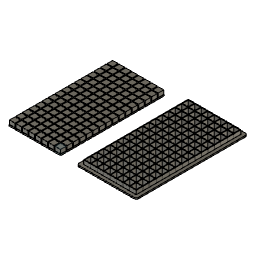
Matriz Altavoz (Autodesk Fusion 360 design; units mm, degrees)
Autodesk Fusion 360 part; units mm, degrees
(part 1 of 2)
sketch "Boceto1" plane through (0, 0, 0) normal (0, 0, 1) x (1, 0, 0)
  line L0 (0, 0) -> (161, 0)
  line L1 (161, 0) -> (161, 81)
  line L2 (161, 81) -> (0, 81)
  line L3 (0, 81) -> (0, 0)
  line L4 (0, 0) -> (0, 1)
  line L5 (0, 1) -> (1, 1)
  line L6 (1, 1) -> (10, 1)
  line L7 (10, 1) -> (10, 10)
  line L8 (10, 10) -> (1, 10)
  line L9 (1, 10) -> (1, 1)
  line L10 (20, 1) -> (20, 10)
  line L11 (20, 10) -> (11, 10)
  line L12 (11, 10) -> (11, 1)
  line L13 (11, 1) -> (20, 1)
  line L14 (30, 1) -> (30, 10)
  line L15 (30, 10) -> (21, 10)
  line L16 (21, 10) -> (21, 1)
  line L17 (21, 1) -> (30, 1)
  line L18 (40, 1) -> (40, 10)
  line L19 (40, 10) -> (31, 10)
  line L20 (31, 10) -> (31, 1)
  line L21 (31, 1) -> (40, 1)
  line L22 (50, 1) -> (50, 10)
  line L23 (50, 10) -> (41, 10)
  line L24 (41, 10) -> (41, 1)
  line L25 (41, 1) -> (50, 1)
  line L26 (60, 1) -> (60, 10)
  line L27 (60, 10) -> (51, 10)
  line L28 (51, 10) -> (51, 1)
  line L29 (51, 1) -> (60, 1)
  line L30 (70, 1) -> (70, 10)
  line L31 (70, 10) -> (61, 10)
  line L32 (61, 10) -> (61, 1)
  line L33 (61, 1) -> (70, 1)
  line L34 (80, 1) -> (80, 10)
  line L35 (80, 10) -> (71, 10)
  line L36 (71, 10) -> (71, 1)
  line L37 (71, 1) -> (80, 1)
  line L38 (90, 1) -> (90, 10)
  line L39 (90, 10) -> (81, 10)
  line L40 (81, 10) -> (81, 1)
  line L41 (81, 1) -> (90, 1)
  line L42 (100, 1) -> (100, 10)
  line L43 (100, 10) -> (91, 10)
  line L44 (91, 10) -> (91, 1)
  line L45 (91, 1) -> (100, 1)
  line L46 (110, 1) -> (110, 10)
  line L47 (110, 10) -> (101, 10)
  line L48 (101, 10) -> (101, 1)
  line L49 (101, 1) -> (110, 1)
  line L50 (120, 1) -> (120, 10)
  line L51 (120, 10) -> (111, 10)
  line L52 (111, 10) -> (111, 1)
  line L53 (111, 1) -> (120, 1)
  line L54 (130, 1) -> (130, 10)
  line L55 (130, 10) -> (121, 10)
  line L56 (121, 10) -> (121, 1)
  line L57 (121, 1) -> (130, 1)
  line L58 (140, 1) -> (140, 10)
  line L59 (140, 10) -> (131, 10)
  line L60 (131, 10) -> (131, 1)
  line L61 (131, 1) -> (140, 1)
  line L62 (150, 1) -> (150, 10)
  line L63 (150, 10) -> (141, 10)
  line L64 (141, 10) -> (141, 1)
  line L65 (141, 1) -> (150, 1)
  line L66 (160, 1) -> (160, 10)
  line L67 (160, 10) -> (151, 10)
  line L68 (151, 10) -> (151, 1)
  line L69 (151, 1) -> (160, 1)
  line L70 (10, 11) -> (10, 20)
  line L71 (10, 20) -> (1, 20)
  line L72 (1, 20) -> (1, 11)
  line L73 (1, 11) -> (10, 11)
  line L74 (20, 11) -> (20, 20)
  line L75 (20, 20) -> (11, 20)
  line L76 (11, 20) -> (11, 11)
  line L77 (11, 11) -> (20, 11)
  line L78 (30, 11) -> (30, 20)
  line L79 (30, 20) -> (21, 20)
  line L80 (21, 20) -> (21, 11)
  line L81 (21, 11) -> (30, 11)
  line L82 (40, 11) -> (40, 20)
  line L83 (40, 20) -> (31, 20)
  line L84 (31, 20) -> (31, 11)
  line L85 (31, 11) -> (40, 11)
  line L86 (50, 11) -> (50, 20)
  line L87 (50, 20) -> (41, 20)
  line L88 (41, 20) -> (41, 11)
  line L89 (41, 11) -> (50, 11)
  line L90 (60, 11) -> (60, 20)
  line L91 (60, 20) -> (51, 20)
  line L92 (51, 20) -> (51, 11)
  line L93 (51, 11) -> (60, 11)
  line L94 (70, 11) -> (70, 20)
  line L95 (70, 20) -> (61, 20)
  line L96 (61, 20) -> (61, 11)
  line L97 (61, 11) -> (70, 11)
  line L98 (80, 11) -> (80, 20)
  line L99 (80, 20) -> (71, 20)
  line L100 (71, 20) -> (71, 11)
  line L101 (71, 11) -> (80, 11)
  line L102 (90, 11) -> (90, 20)
  line L103 (90, 20) -> (81, 20)
  line L104 (81, 20) -> (81, 11)
  line L105 (81, 11) -> (90, 11)
  line L106 (100, 11) -> (100, 20)
  line L107 (100, 20) -> (91, 20)
  line L108 (91, 20) -> (91, 11)
  line L109 (91, 11) -> (100, 11)
  line L110 (110, 11) -> (110, 20)
  line L111 (110, 20) -> (101, 20)
  line L112 (101, 20) -> (101, 11)
  line L113 (101, 11) -> (110, 11)
  line L114 (120, 11) -> (120, 20)
  line L115 (120, 20) -> (111, 20)
  line L116 (111, 20) -> (111, 11)
  line L117 (111, 11) -> (120, 11)
  line L118 (130, 11) -> (130, 20)
  line L119 (130, 20) -> (121, 20)
  line L120 (121, 20) -> (121, 11)
  line L121 (121, 11) -> (130, 11)
  line L122 (140, 11) -> (140, 20)
  line L123 (140, 20) -> (131, 20)
  line L124 (131, 20) -> (131, 11)
  line L125 (131, 11) -> (140, 11)
  line L126 (150, 11) -> (150, 20)
  line L127 (150, 20) -> (141, 20)
  line L128 (141, 20) -> (141, 11)
  line L129 (141, 11) -> (150, 11)
  line L130 (160, 11) -> (160, 20)
  line L131 (160, 20) -> (151, 20)
  line L132 (151, 20) -> (151, 11)
  line L133 (151, 11) -> (160, 11)
  line L134 (10, 21) -> (10, 30)
  line L135 (10, 30) -> (1, 30)
  line L136 (1, 30) -> (1, 21)
  line L137 (1, 21) -> (10, 21)
  line L138 (20, 21) -> (20, 30)
  line L139 (20, 30) -> (11, 30)
  line L140 (11, 30) -> (11, 21)
  line L141 (11, 21) -> (20, 21)
  line L142 (30, 21) -> (30, 30)
  line L143 (30, 30) -> (21, 30)
  line L144 (21, 30) -> (21, 21)
  line L145 (21, 21) -> (30, 21)
  line L146 (40, 21) -> (40, 30)
  line L147 (40, 30) -> (31, 30)
  line L148 (31, 30) -> (31, 21)
  line L149 (31, 21) -> (40, 21)
  line L150 (50, 21) -> (50, 30)
  line L151 (50, 30) -> (41, 30)
  line L152 (41, 30) -> (41, 21)
  line L153 (41, 21) -> (50, 21)
  line L154 (60, 21) -> (60, 30)
  line L155 (60, 30) -> (51, 30)
  line L156 (51, 30) -> (51, 21)
  line L157 (51, 21) -> (60, 21)
  line L158 (70, 21) -> (70, 30)
  line L159 (70, 30) -> (61, 30)
  line L160 (61, 30) -> (61, 21)
  line L161 (61, 21) -> (70, 21)
  line L162 (80, 21) -> (80, 30)
  line L163 (80, 30) -> (71, 30)
  line L164 (71, 30) -> (71, 21)
  line L165 (71, 21) -> (80, 21)
  line L166 (90, 21) -> (90, 30)
  line L167 (90, 30) -> (81, 30)
  line L168 (81, 30) -> (81, 21)
  line L169 (81, 21) -> (90, 21)
  line L170 (100, 21) -> (100, 30)
  line L171 (100, 30) -> (91, 30)
  line L172 (91, 30) -> (91, 21)
  line L173 (91, 21) -> (100, 21)
  line L174 (110, 21) -> (110, 30)
  line L175 (110, 30) -> (101, 30)
  line L176 (101, 30) -> (101, 21)
  line L177 (101, 21) -> (110, 21)
  line L178 (120, 21) -> (120, 30)
  line L179 (120, 30) -> (111, 30)
  line L180 (111, 30) -> (111, 21)
  line L181 (111, 21) -> (120, 21)
  line L182 (130, 21) -> (130, 30)
  line L183 (130, 30) -> (121, 30)
  line L184 (121, 30) -> (121, 21)
  line L185 (121, 21) -> (130, 21)
  line L186 (140, 21) -> (140, 30)
  line L187 (140, 30) -> (131, 30)
  line L188 (131, 30) -> (131, 21)
  line L189 (131, 21) -> (140, 21)
  line L190 (150, 21) -> (150, 30)
  line L191 (150, 30) -> (141, 30)
  line L192 (141, 30) -> (141, 21)
  line L193 (141, 21) -> (150, 21)
  line L194 (160, 21) -> (160, 30)
  line L195 (160, 30) -> (151, 30)
  line L196 (151, 30) -> (151, 21)
  line L197 (151, 21) -> (160, 21)
  line L198 (10, 31) -> (10, 40)
  line L199 (10, 40) -> (1, 40)
  line L200 (1, 40) -> (1, 31)
  line L201 (1, 31) -> (10, 31)
  line L202 (20, 31) -> (20, 40)
  line L203 (20, 40) -> (11, 40)
  line L204 (11, 40) -> (11, 31)
  line L205 (11, 31) -> (20, 31)
  line L206 (30, 31) -> (30, 40)
  line L207 (30, 40) -> (21, 40)
  line L208 (21, 40) -> (21, 31)
  line L209 (21, 31) -> (30, 31)
  line L210 (40, 31) -> (40, 40)
  line L211 (40, 40) -> (31, 40)
  line L212 (31, 40) -> (31, 31)
  line L213 (31, 31) -> (40, 31)
  line L214 (50, 31) -> (50, 40)
  line L215 (50, 40) -> (41, 40)
  line L216 (41, 40) -> (41, 31)
  line L217 (41, 31) -> (50, 31)
  line L218 (60, 31) -> (60, 40)
  line L219 (60, 40) -> (51, 40)
  line L220 (51, 40) -> (51, 31)
  line L221 (51, 31) -> (60, 31)
  line L222 (70, 31) -> (70, 40)
  line L223 (70, 40) -> (61, 40)
  line L224 (61, 40) -> (61, 31)
  line L225 (61, 31) -> (70, 31)
  line L226 (80, 31) -> (80, 40)
  line L227 (80, 40) -> (71, 40)
  line L228 (71, 40) -> (71, 31)
  line L229 (71, 31) -> (80, 31)
  line L230 (90, 31) -> (90, 40)
  line L231 (90, 40) -> (81, 40)
  line L232 (81, 40) -> (81, 31)
  line L233 (81, 31) -> (90, 31)
  line L234 (100, 31) -> (100, 40)
  line L235 (100, 40) -> (91, 40)
  line L236 (91, 40) -> (91, 31)
  line L237 (91, 31) -> (100, 31)
  line L238 (110, 31) -> (110, 40)
  line L239 (110, 40) -> (101, 40)
  line L240 (101, 40) -> (101, 31)
  line L241 (101, 31) -> (110, 31)
  line L242 (120, 31) -> (120, 40)
  line L243 (120, 40) -> (111, 40)
  line L244 (111, 40) -> (111, 31)
  line L245 (111, 31) -> (120, 31)
  line L246 (130, 31) -> (130, 40)
  line L247 (130, 40) -> (121, 40)
  line L248 (121, 40) -> (121, 31)
  line L249 (121, 31) -> (130, 31)
  line L250 (140, 31) -> (140, 40)
  line L251 (140, 40) -> (131, 40)
  line L252 (131, 40) -> (131, 31)
  line L253 (131, 31) -> (140, 31)
  line L254 (150, 31) -> (150, 40)
  line L255 (150, 40) -> (141, 40)
  line L256 (141, 40) -> (141, 31)
  line L257 (141, 31) -> (150, 31)
  line L258 (160, 31) -> (160, 40)
  line L259 (160, 40) -> (151, 40)
  line L260 (151, 40) -> (151, 31)
  line L261 (151, 31) -> (160, 31)
  line L262 (10, 41) -> (10, 50)
  line L263 (10, 50) -> (1, 50)
  line L264 (1, 50) -> (1, 41)
  line L265 (1, 41) -> (10, 41)
  line L266 (20, 41) -> (20, 50)
  line L267 (20, 50) -> (11, 50)
  line L268 (11, 50) -> (11, 41)
  line L269 (11, 41) -> (20, 41)
  line L270 (30, 41) -> (30, 50)
  line L271 (30, 50) -> (21, 50)
  line L272 (21, 50) -> (21, 41)
  line L273 (21, 41) -> (30, 41)
  line L274 (40, 41) -> (40, 50)
  line L275 (40, 50) -> (31, 50)
  line L276 (31, 50) -> (31, 41)
  line L277 (31, 41) -> (40, 41)
  line L278 (50, 41) -> (50, 50)
  line L279 (50, 50) -> (41, 50)
  line L280 (41, 50) -> (41, 41)
  line L281 (41, 41) -> (50, 41)
  line L282 (60, 41) -> (60, 50)
  line L283 (60, 50) -> (51, 50)
  line L284 (51, 50) -> (51, 41)
  line L285 (51, 41) -> (60, 41)
  line L286 (70, 41) -> (70, 50)
  line L287 (70, 50) -> (61, 50)
  line L288 (61, 50) -> (61, 41)
  line L289 (61, 41) -> (70, 41)
  line L290 (80, 41) -> (80, 50)
  line L291 (80, 50) -> (71, 50)
  line L292 (71, 50) -> (71, 41)
  line L293 (71, 41) -> (80, 41)
  line L294 (90, 41) -> (90, 50)
  line L295 (90, 50) -> (81, 50)
  line L296 (81, 50) -> (81, 41)
  line L297 (81, 41) -> (90, 41)
  line L298 (100, 41) -> (100, 50)
  line L299 (100, 50) -> (91, 50)
  line L300 (91, 50) -> (91, 41)
  line L301 (91, 41) -> (100, 41)
  line L302 (110, 41) -> (110, 50)
  line L303 (110, 50) -> (101, 50)
  line L304 (101, 50) -> (101, 41)
  line L305 (101, 41) -> (110, 41)
  line L306 (120, 41) -> (120, 50)
  line L307 (120, 50) -> (111, 50)
  line L308 (111, 50) -> (111, 41)
  line L309 (111, 41) -> (120, 41)
  line L310 (130, 41) -> (130, 50)
  line L311 (130, 50) -> (121, 50)
  line L312 (121, 50) -> (121, 41)
  line L313 (121, 41) -> (130, 41)
  line L314 (140, 41) -> (140, 50)
  line L315 (140, 50) -> (131, 50)
  line L316 (131, 50) -> (131, 41)
  line L317 (131, 41) -> (140, 41)
  line L318 (150, 41) -> (150, 50)
  line L319 (150, 50) -> (141, 50)
  line L320 (141, 50) -> (141, 41)
  line L321 (141, 41) -> (150, 41)
  line L322 (160, 41) -> (160, 50)
  line L323 (160, 50) -> (151, 50)
  line L324 (151, 50) -> (151, 41)
  line L325 (151, 41) -> (160, 41)
  line L326 (10, 51) -> (10, 60)
  line L327 (10, 60) -> (1, 60)
  line L328 (1, 60) -> (1, 51)
  line L329 (1, 51) -> (10, 51)
  line L330 (20, 51) -> (20, 60)
  line L331 (20, 60) -> (11, 60)
  line L332 (11, 60) -> (11, 51)
  line L333 (11, 51) -> (20, 51)
  line L334 (30, 51) -> (30, 60)
  line L335 (30, 60) -> (21, 60)
  line L336 (21, 60) -> (21, 51)
  line L337 (21, 51) -> (30, 51)
  line L338 (40, 51) -> (40, 60)
  line L339 (40, 60) -> (31, 60)
  line L340 (31, 60) -> (31, 51)
  line L341 (31, 51) -> (40, 51)
  line L342 (50, 51) -> (50, 60)
  line L343 (50, 60) -> (41, 60)
  line L344 (41, 60) -> (41, 51)
  line L345 (41, 51) -> (50, 51)
  line L346 (60, 51) -> (60, 60)
  line L347 (60, 60) -> (51, 60)
  line L348 (51, 60) -> (51, 51)
  line L349 (51, 51) -> (60, 51)
  line L350 (70, 51) -> (70, 60)
  line L351 (70, 60) -> (61, 60)
  line L352 (61, 60) -> (61, 51)
  line L353 (61, 51) -> (70, 51)
  line L354 (80, 51) -> (80, 60)
  line L355 (80, 60) -> (71, 60)
  line L356 (71, 60) -> (71, 51)
  line L357 (71, 51) -> (80, 51)
  line L358 (90, 51) -> (90, 60)
  line L359 (90, 60) -> (81, 60)
  line L360 (81, 60) -> (81, 51)
  line L361 (81, 51) -> (90, 51)
  line L362 (100, 51) -> (100, 60)
  line L363 (100, 60) -> (91, 60)
  line L364 (91, 60) -> (91, 51)
  line L365 (91, 51) -> (100, 51)
  line L366 (110, 51) -> (110, 60)
  line L367 (110, 60) -> (101, 60)
  line L368 (101, 60) -> (101, 51)
  line L369 (101, 51) -> (110, 51)
  line L370 (120, 51) -> (120, 60)
  line L371 (120, 60) -> (111, 60)
  line L372 (111, 60) -> (111, 51)
  line L373 (111, 51) -> (120, 51)
  line L374 (130, 51) -> (130, 60)
  line L375 (130, 60) -> (121, 60)
  line L376 (121, 60) -> (121, 51)
  line L377 (121, 51) -> (130, 51)
  line L378 (140, 51) -> (140, 60)
  line L379 (140, 60) -> (131, 60)
  line L380 (131, 60) -> (131, 51)
  line L381 (131, 51) -> (140, 51)
  line L382 (150, 51) -> (150, 60)
  line L383 (150, 60) -> (141, 60)
  line L384 (141, 60) -> (141, 51)
  line L385 (141, 51) -> (150, 51)
  line L386 (160, 51) -> (160, 60)
  line L387 (160, 60) -> (151, 60)
  line L388 (151, 60) -> (151, 51)
  line L389 (151, 51) -> (160, 51)
  line L390 (10, 61) -> (10, 70)
  line L391 (10, 70) -> (1, 70)
  line L392 (1, 70) -> (1, 61)
  line L393 (1, 61) -> (10, 61)
  line L394 (20, 61) -> (20, 70)
  line L395 (20, 70) -> (11, 70)
  line L396 (11, 70) -> (11, 61)
  line L397 (11, 61) -> (20, 61)
  line L398 (30, 61) -> (30, 70)
  line L399 (30, 70) -> (21, 70)
  line L400 (21, 70) -> (21, 61)
  line L401 (21, 61) -> (30, 61)
  line L402 (40, 61) -> (40, 70)
  line L403 (40, 70) -> (31, 70)
  line L404 (31, 70) -> (31, 61)
  line L405 (31, 61) -> (40, 61)
  line L406 (50, 61) -> (50, 70)
  line L407 (50, 70) -> (41, 70)
  line L408 (41, 70) -> (41, 61)
  line L409 (41, 61) -> (50, 61)
  line L410 (60, 61) -> (60, 70)
  line L411 (60, 70) -> (51, 70)
  line L412 (51, 70) -> (51, 61)
  line L413 (51, 61) -> (60, 61)
  line L414 (70, 61) -> (70, 70)
  line L415 (70, 70) -> (61, 70)
  line L416 (61, 70) -> (61, 61)
  line L417 (61, 61) -> (70, 61)
  line L418 (80, 61) -> (80, 70)
  line L419 (80, 70) -> (71, 70)
  line L420 (71, 70) -> (71, 61)
  line L421 (71, 61) -> (80, 61)
  line L422 (90, 61) -> (90, 70)
  line L423 (90, 70) -> (81, 70)
  line L424 (81, 70) -> (81, 61)
  line L425 (81, 61) -> (90, 61)
  line L426 (100, 61) -> (100, 70)
  line L427 (100, 70) -> (91, 70)
  line L428 (91, 70) -> (91, 61)
  line L429 (91, 61) -> (100, 61)
  line L430 (110, 61) -> (110, 70)
  line L431 (110, 70) -> (101, 70)
  line L432 (101, 70) -> (101, 61)
  line L433 (101, 61) -> (110, 61)
  line L434 (120, 61) -> (120, 70)
  line L435 (120, 70) -> (111, 70)
  line L436 (111, 70) -> (111, 61)
  line L437 (111, 61) -> (120, 61)
  line L438 (130, 61) -> (130, 70)
  line L439 (130, 70) -> (121, 70)
  line L440 (121, 70) -> (121, 61)
  line L441 (121, 61) -> (130, 61)
  line L442 (140, 61) -> (140, 70)
  line L443 (140, 70) -> (131, 70)
  line L444 (131, 70) -> (131, 61)
  line L445 (131, 61) -> (140, 61)
  line L446 (150, 61) -> (150, 70)
  line L447 (150, 70) -> (141, 70)
  line L448 (141, 70) -> (141, 61)
  line L449 (141, 61) -> (150, 61)
  line L450 (160, 61) -> (160, 70)
  line L451 (160, 70) -> (151, 70)
  line L452 (151, 70) -> (151, 61)
  line L453 (151, 61) -> (160, 61)
  line L454 (10, 71) -> (10, 80)
  line L455 (10, 80) -> (1, 80)
  line L456 (1, 80) -> (1, 71)
  line L457 (1, 71) -> (10, 71)
  line L458 (20, 71) -> (20, 80)
  line L459 (20, 80) -> (11, 80)
  line L460 (11, 80) -> (11, 71)
  line L461 (11, 71) -> (20, 71)
  line L462 (30, 71) -> (30, 80)
  line L463 (30, 80) -> (21, 80)
  line L464 (21, 80) -> (21, 71)
  line L465 (21, 71) -> (30, 71)
  line L466 (40, 71) -> (40, 80)
  line L467 (40, 80) -> (31, 80)
  line L468 (31, 80) -> (31, 71)
  line L469 (31, 71) -> (40, 71)
  line L470 (50, 71) -> (50, 80)
  line L471 (50, 80) -> (41, 80)
  line L472 (41, 80) -> (41, 71)
  line L473 (41, 71) -> (50, 71)
  line L474 (60, 71) -> (60, 80)
  line L475 (60, 80) -> (51, 80)
  line L476 (51, 80) -> (51, 71)
  line L477 (51, 71) -> (60, 71)
  line L478 (70, 71) -> (70, 80)
  line L479 (70, 80) -> (61, 80)
  line L480 (61, 80) -> (61, 71)
  line L481 (61, 71) -> (70, 71)
  line L482 (80, 71) -> (80, 80)
  line L483 (80, 80) -> (71, 80)
  line L484 (71, 80) -> (71, 71)
  line L485 (71, 71) -> (80, 71)
  line L486 (90, 71) -> (90, 80)
  line L487 (90, 80) -> (81, 80)
  line L488 (81, 80) -> (81, 71)
  line L489 (81, 71) -> (90, 71)
  line L490 (100, 71) -> (100, 80)
  line L491 (100, 80) -> (91, 80)
  line L492 (91, 80) -> (91, 71)
  line L493 (91, 71) -> (100, 71)
  line L494 (110, 71) -> (110, 80)
  line L495 (110, 80) -> (101, 80)
  line L496 (101, 80) -> (101, 71)
  line L497 (101, 71) -> (110, 71)
  line L498 (120, 71) -> (120, 80)
  line L499 (120, 80) -> (111, 80)
  line L500 (111, 80) -> (111, 71)
  line L501 (111, 71) -> (120, 71)
  line L502 (130, 71) -> (130, 80)
  line L503 (130, 80) -> (121, 80)
  line L504 (121, 80) -> (121, 71)
  line L505 (121, 71) -> (130, 71)
  line L506 (140, 71) -> (140, 80)
  line L507 (140, 80) -> (131, 80)
  line L508 (131, 80) -> (131, 71)
  line L509 (131, 71) -> (140, 71)
  line L510 (150, 71) -> (150, 80)
  line L511 (150, 80) -> (141, 80)
  line L512 (141, 80) -> (141, 71)
  line L513 (141, 71) -> (150, 71)
  line L514 (160, 71) -> (160, 80)
  line L515 (160, 80) -> (151, 80)
  line L516 (151, 80) -> (151, 71)
  line L517 (151, 71) -> (160, 71)
  dimension "d1" = 161
  dimension "d2" = 81
  dimension "d3" = 1
  dimension "d4" = 9
  dimension "d5" = 9
  dimension "d8" = 150
  dimension "d9" = 70
  constraint horizontal L0
  constraint vertical L1
  constraint horizontal L2
  constraint vertical L3
  constraint coincident L0.start L3.end
  constraint vertical L4
  constraint perpendicular L3 L5
  constraint horizontal L6
  constraint vertical L7
  constraint horizontal L8
  constraint vertical L9
  measures "d1" distance of L0.start L0.end
  measures "d2" distance of L0.start L2.end
  measures "d3" distance of L0.start L4.end
  measures "d4" distance of L5.end L6.end
  measures "d5" distance of L5.end L8.end
extrude "Extruir1" add sketch "Boceto1" along normal blind 10 makes body 1
sketch "Boceto2" plane through (0, 0, 0) normal (0, 0, 1) x (1, 0, 0)
sketch "Boceto3" plane through (0, 0, 0) normal (0, 0, 1) x (1, 0, 0)
  line L0 (0, 85) -> (8.8, 85)
  line L1 (8.8, 85) -> (8.8, 93.8)
  line L2 (8.8, 93.8) -> (0, 93.8)
  line L3 (0, 93.8) -> (0, 85)
  dimension "d12" = 8.8
  dimension "d13" = 8.8
  constraint horizontal L0
  constraint vertical L1
  constraint horizontal L2
  constraint vertical L3
  measures "d12" distance of L0.start L0.end
  measures "d13" distance of L0.start L2.end
extrude "Extruir2" add sketch "Boceto3" along normal blind 1 separate body makes body 2
sketch "Boceto4" plane through (0, 0, 1) normal (0, 0, 1) x (-1, 0, 0)
  line L0 (0, -93.8) -> (0, -85)
  line L1 (0, -85) -> (-8.8, -85)
  line L2 (-8.8, -85) -> (-8.8, -93.8)
  line L3 (-8.8, -93.8) -> (0, -93.8)
  line L4 (0, -93.8) -> (-8.8, -93.8)
  line L5 (-8.8, -93.8) -> (-8.8, -85)
  line L6 (-8.8, -85) -> (0, -85)
  line L7 (0, -85) -> (0, -93.8)
  line L8 (0, -93.8) -> (-1, -93.8)
  line L9 (-1, -93.8) -> (-1, -92.8)
  line L10 (-8.8, -85) -> (-7.8, -85)
  line L11 (-7.8, -85) -> (-7.8, -86)
  line L12 (-7.8, -86) -> (-1, -86)
  line L13 (-1, -86) -> (-1, -92.8)
  line L14 (-1, -92.8) -> (-7.8, -92.8)
  line L15 (-7.8, -92.8) -> (-7.8, -86)
  dimension "d16" = 1
  constraint horizontal L4
  constraint vertical L5
  constraint horizontal L6
  constraint vertical L7
  constraint coincident L1.end L2.start
  constraint coincident L0.start L3.end
  constraint coincident L4 L8.end
  constraint perpendicular L4 L9
  constraint perpendicular L5 L10
  constraint perpendicular L10 L11
  constraint horizontal L12
  constraint vertical L13
  constraint horizontal L14
  constraint vertical L15
  measures "d16" distance of L1.end L10.end
extrude "Extruir3" add sketch "Boceto4" along normal blind 11 contours L0 L1 L3 L4 L6 L7 L8 L9 L11 L12 L13 | L1 L2 L3 L4 L5 L6 L9 L10 L11 L14 L15 bodies 2
extrude "Extruir4" add 1 faces at (3.2667, 90.5333, 1) along direction (0, 0, 1) blind 2 on bodies 2 bodies 2
sketch "Boceto5" plane through (0, 0, 12) normal (0, 0, 1) x (-1, 0, 0)
  line L0 (-1, -92.8) -> (-7.8, -92.8)
  line L1 (-7.8, -92.8) -> (-7.8, -86)
  line L2 (-7.8, -86) -> (-1, -86)
  line L3 (-1, -86) -> (-1, -92.8)
  line L4 (-8.8, -85) -> (-8.8, -93.8)
  line L5 (-8.8, -93.8) -> (0, -93.8)
  line L6 (0, -93.8) -> (0, -85)
  line L7 (0, -85) -> (-8.8, -85)
  line L8 (0, -93.8) -> (-0.1, -93.8)
  line L9 (-0.1, -93.8) -> (-0.1, -93.7)
  line L10 (-0.1, -93.7) -> (-8.7, -93.7)
  line L11 (-8.7, -93.7) -> (-8.7, -85.1)
  line L12 (-8.7, -85.1) -> (-0.1, -85.1)
  line L13 (-0.1, -85.1) -> (-0.1, -93.7)
  dimension "d21" = 0.1
  constraint coincident L5.end L6.start
  constraint horizontal L8
  constraint perpendicular L5 L9
  constraint horizontal L10
  constraint vertical L11
  constraint horizontal L12
  constraint vertical L13
  measures "d21" distance of L5.end L8.end
extrude "Extruir5" cut sketch "Boceto5" against normal blind 20 contours L4 L5 L6 L7 L8 bodies 2
sketch "Boceto6" plane through (0, 0, 12) normal (0, 0, 1) x (-1, 0, 0)
  line L0 (-0.1, -93.7) -> (-0.1, -85.1)
  line L1 (-0.1, -85.1) -> (-8.7, -85.1)
  line L2 (-8.7, -85.1) -> (-8.7, -93.7)
  line L3 (-8.7, -93.7) -> (-0.1, -93.7)
  line L4 (-1, -92.8) -> (-7.8, -92.8)
  line L5 (-7.8, -92.8) -> (-7.8, -86)
  line L6 (-7.8, -86) -> (-1, -86)
  line L7 (-1, -86) -> (-1, -92.8)
  line L8 (-1, -92.8) -> (-1.2, -92.8)
  line L9 (-1.2, -92.8) -> (-1.2, -92.6)
  line L10 (-7.8, -86) -> (-7.6, -86)
  line L11 (-7.6, -86) -> (-7.6, -86.2)
  line L12 (-7.6, -86.2) -> (-1.2, -86.2)
  line L13 (-1.2, -86.2) -> (-1.2, -92.6)
  line L14 (-1.2, -92.6) -> (-7.6, -92.6)
  line L15 (-7.6, -92.6) -> (-7.6, -86.2)
  constraint coincident L4.start L7.end
  constraint coincident L4 L8.end
  constraint perpendicular L8 L9
  constraint coincident L5.end L6.start
  constraint coincident L6 L10.end
  constraint perpendicular L5 L10
  constraint perpendicular L10 L11
  constraint horizontal L12
  constraint vertical L13
  constraint horizontal L14
  constraint vertical L15
extrude "Extruir6" add sketch "Boceto6" against normal blind 11 contours L4 L6 L7 L8 L9 L11 L12 L13 | L4 L5 L6 L9 L10 L11 L14 L15 bodies 2
sketch "Boceto7" plane through (0, 0, 0) normal (0, 0, -1) x (1, 0, 0)
  line L0 (0.1, -85.1) -> (0.1, -93.7)
  line L1 (0.1, -93.7) -> (8.7, -93.7)
  line L2 (8.7, -93.7) -> (8.7, -85.1)
  line L3 (8.7, -85.1) -> (0.1, -85.1)
sketch "Boceto8" plane through (0, 0, 0) normal (0, 0, -1) x (1, 0, 0)
  line L0 (0.1, -85.1) -> (-0.2, -85.1)
  line L1 (-0.2, -85.1) -> (-0.2, -84.8)
  line L2 (8.7, -93.7) -> (8.7, -94)
  line L3 (8.7, -94) -> (9, -94)
  line L4 (9, -94) -> (-0.2, -94)
  line L5 (-0.2, -94) -> (-0.2, -84.8)
  line L6 (-0.2, -84.8) -> (9, -84.8)
  line L7 (9, -84.8) -> (9, -94)
  dimension "d26" = 0.3
  constraint horizontal L0
  constraint perpendicular L0 L1
  constraint vertical L2
  constraint perpendicular L2 L3
  constraint horizontal L4
  constraint vertical L5
  constraint horizontal L6
  constraint vertical L7
  measures "d26" distance of L0.start L0.end
extrude "Extruir7" add sketch "Boceto8" against normal blind 2 bodies 2
sketch "Boceto9" plane through (0, 0, 12) normal (0, 0, 1) x (-1, 0, 0)
  line L0 (-1.2, -92.6) -> (-7.6, -92.6)
  line L1 (-7.6, -92.6) -> (-7.6, -86.2)
  line L2 (-7.6, -86.2) -> (-1.2, -86.2)
  line L3 (-1.2, -86.2) -> (-1.2, -92.6)
  line L4 (-0.1, -93.7) -> (-0.1, -85.1)
  line L5 (-0.1, -85.1) -> (-8.7, -85.1)
  line L6 (-8.7, -85.1) -> (-8.7, -93.7)
  line L7 (-8.7, -93.7) -> (-0.1, -93.7)
  line L8 (-0.1, -93.7) -> (-0.2, -93.7)
  line L9 (-0.2, -93.7) -> (-0.2, -93.6)
  line L10 (-8.7, -85.1) -> (-8.6, -85.1)
  line L11 (-8.6, -85.1) -> (-8.6, -85.2)
  line L12 (-8.6, -85.2) -> (-0.2, -85.2)
  line L13 (-0.2, -85.2) -> (-0.2, -93.6)
  line L14 (-0.2, -93.6) -> (-8.6, -93.6)
  line L15 (-8.6, -93.6) -> (-8.6, -85.2)
  constraint coincident L4.start L7.end
  constraint coincident L7 L8.end
  constraint perpendicular L8 L9
  constraint coincident L5.end L6.start
  constraint coincident L5 L10.end
  constraint perpendicular L6 L10
  constraint perpendicular L5 L11
  constraint horizontal L12
  constraint vertical L13
  constraint horizontal L14
  constraint vertical L15
extrude "Extruir8" cut sketch "Boceto9" against normal blind 10 contours L4 L5 L7 L8 L9 L11 L12 L13 | L5 L6 L7 L9 L10 L11 L14 L15 bodies 2
sketch "Boceto10" plane through (0, 0, 12) normal (0, 0, 1) x (-1, 0, 0)
  line L0 (-8.6, -85.2) -> (-8.6, -93.6)
  line L1 (-8.6, -93.6) -> (-0.2, -93.6)
  line L2 (-0.2, -93.6) -> (-0.2, -85.2)
  line L3 (-0.2, -85.2) -> (-8.6, -85.2)
  line L4 (-1.2, -92.6) -> (-7.6, -92.6)
  line L5 (-7.6, -92.6) -> (-7.6, -86.2)
  line L6 (-7.6, -86.2) -> (-1.2, -86.2)
  line L7 (-1.2, -86.2) -> (-1.2, -92.6)
  line L8 (-1.2, -92.6) -> (-7.6, -92.6)
  line L9 (-7.6, -92.6) -> (-7.6, -86.2)
  line L10 (-7.6, -86.2) -> (-1.2, -86.2)
  line L11 (-1.2, -86.2) -> (-1.2, -92.6)
  constraint horizontal L8
  constraint vertical L9
  constraint horizontal L10
  constraint vertical L11
  constraint coincident L5.end L6.start
  constraint coincident L4.start L7.end
extrude "Extruir9" add sketch "Boceto10" against normal blind 10 contours L4 L5 L6 L7 L8 L9 L10 L11 bodies 2
sketch "Boceto11" plane through (0, 0, 12) normal (0, 0, 1) x (-1, 0, 0)
  line L0 (-8.6, -85.2) -> (-8.6, -93.6)
  line L1 (-8.6, -93.6) -> (-0.2, -93.6)
  line L2 (-0.2, -93.6) -> (-0.2, -85.2)
  line L3 (-0.2, -85.2) -> (-8.6, -85.2)
  line L4 (-0.2, -93.6) -> (-8.6, -93.6)
  line L5 (-8.6, -93.6) -> (-8.6, -85.2)
  line L6 (-8.6, -85.2) -> (-0.2, -85.2)
  line L7 (-0.2, -85.2) -> (-0.2, -93.6)
  constraint horizontal L4
  constraint vertical L5
  constraint horizontal L6
  constraint vertical L7
  constraint coincident L0.start L3.end
  constraint coincident L1.end L2.start
extrude "Extruir10" cut sketch "Boceto11" against normal blind 5 bodies 2
extrude "Extruir11" add 1 faces at (5.8, 88, 7) along direction (0, 0, 1) blind 1 on bodies 2 bodies 2
sketch "Boceto12" plane through (0, 0, 8) normal (0, 0, 1) x (-1, 0, 0)
  line L0 (-0.2, -85.2) -> (-8.6, -85.2)
  line L1 (-8.6, -85.2) -> (-8.6, -93.6)
  line L2 (-8.6, -93.6) -> (-0.2, -93.6)
  line L3 (-0.2, -93.6) -> (-0.2, -85.2)
  line L4 (-0.2, -93.6) -> (-0.15, -93.6)
  line L5 (-0.15, -93.6) -> (-0.15, -93.65)
  line L6 (-8.6, -85.2) -> (-8.6, -85.15)
  line L7 (-8.6, -85.15) -> (-8.65, -85.15)
  line L8 (-8.65, -85.15) -> (-0.15, -85.15)
  line L9 (-0.15, -85.15) -> (-0.15, -93.65)
  line L10 (-0.15, -93.65) -> (-8.65, -93.65)
  line L11 (-8.65, -93.65) -> (-8.65, -85.15)
  constraint coincident L2.end L3.start
  constraint perpendicular L3 L4
  constraint perpendicular L4 L5
  constraint coincident L0.end L1.start
  constraint perpendicular L0 L6
  constraint perpendicular L6 L7
  constraint horizontal L8
  constraint vertical L9
  constraint horizontal L10
  constraint vertical L11
extrude "Extruir12" add sketch "Boceto12" against normal blind 6 contours L0 L3 L4 L6 L8 L9 | L1 L2 L4 L5 L6 L7 L8 L9 L10 L11 bodies 2
sketch "Boceto13" plane through (0, 0, 8) normal (0, 0, 1) x (-1, 0, 0)
  line L0 (-8.65, -93.65) -> (-0.15, -93.65)
  line L1 (-0.15, -93.65) -> (-0.15, -85.15)
  line L2 (-0.15, -85.15) -> (-8.65, -85.15)
  line L3 (-8.65, -85.15) -> (-8.65, -93.65)
pattern_linear "Patrón R1" count 16 spacing 10 along (0, 1, 0) count 8 spacing 10 along (-1, 0, 0) of bodies 2 makes body 3 at (2.8667, 97.8667, 0) makes body 4 at (2.8667, 107.8667, 0) makes body 5 at (2.8667, 117.8667, 0) makes body 6 at (2.8667, 127.8667, 0) makes body 7 at (2.8667, 137.8667, 0) makes body 8 at (2.8667, 147.8667, 0) makes body 9 at (2.8667, 157.8667, 0) makes body 10 at (2.8667, 167.8667, 0) makes body 11 at (2.8667, 177.8667, 0) makes body 12 at (2.8667, 187.8667, 0) makes body 13 at (2.8667, 197.8667, 0) makes body 14 at (2.8667, 207.8667, 0) makes body 15 at (2.8667, 217.8667, 0) makes body 16 at (2.8667, 227.8667, 0) makes body 17 at (2.8667, 237.8667, 0) makes body 18 at (-7.1333, 87.8667, 0) makes body 19 at (-7.1333, 97.8667, 0) makes body 20 at (-7.1333, 107.8667, 0) makes body 21 at (-7.1333, 117.8667, 0) makes body 22 at (-7.1333, 127.8667, 0) makes body 23 at (-7.1333, 137.8667, 0) makes body 24 at (-7.1333, 147.8667, 0) makes body 25 at (-7.1333, 157.8667, 0) makes body 26 at (-7.1333, 167.8667, 0) makes body 27 at (-7.1333, 177.8667, 0) makes body 28 at (-7.1333, 187.8667, 0) makes body 29 at (-7.1333, 197.8667, 0) makes body 30 at (-7.1333, 207.8667, 0) makes body 31 at (-7.1333, 217.8667, 0) makes body 32 at (-7.1333, 227.8667, 0) makes body 33 at (-7.1333, 237.8667, 0) makes body 34 at (-17.1333, 90.9333, 0) makes body 35 at (-17.1333, 100.9333, 0) makes body 36 at (-17.1333, 110.9333, 0) makes body 37 at (-17.1333, 120.9333, 0) makes body 38 at (-17.1333, 130.9333, 0) makes body 39 at (-17.1333, 140.9333, 0) makes body 40 at (-17.1333, 150.9333, 0) makes body 41 at (-17.1333, 160.9333, 0) makes body 42 at (-17.1333, 170.9333, 0) makes body 43 at (-17.1333, 180.9333, 0) makes body 44 at (-17.1333, 190.9333, 0) makes body 45 at (-17.1333, 200.9333, 0) makes body 46 at (-17.1333, 210.9333, 0) makes body 47 at (-17.1333, 220.9333, 0) makes body 48 at (-17.1333, 230.9333, 0) makes body 49 at (-17.1333, 240.9333, 0) makes body 50 at (-27.1333, 87.8667, 0) makes body 51 at (-27.1333, 97.8667, 0) makes body 52 at (-27.1333, 107.8667, 0) makes body 53 at (-27.1333, 117.8667, 0) makes body 54 at (-27.1333, 127.8667, 0) makes body 55 at (-27.1333, 137.8667, 0) makes body 56 at (-27.1333, 147.8667, 0) makes body 57 at (-27.1333, 157.8667, 0) makes body 58 at (-27.1333, 167.8667, 0) makes body 59 at (-27.1333, 177.8667, 0) makes body 60 at (-27.1333, 187.8667, 0) makes body 61 at (-27.1333, 197.8667, 0) makes body 62 at (-27.1333, 207.8667, 0) makes body 63 at (-27.1333, 217.8667, 0) makes body 64 at (-27.1333, 227.8667, 0) makes body 65 at (-27.1333, 237.8667, 0) makes body 66 at (-37.1333, 90.9333, 0) makes body 67 at (-37.1333, 100.9333, 0) makes body 68 at (-37.1333, 110.9333, 0) makes body 69 at (-37.1333, 120.9333, 0) makes body 70 at (-37.1333, 130.9333, 0) makes body 71 at (-37.1333, 140.9333, 0) makes body 72 at (-37.1333, 150.9333, 0) makes body 73 at (-37.1333, 160.9333, 0) makes body 74 at (-37.1333, 170.9333, 0) makes body 75 at (-37.1333, 180.9333, 0) makes body 76 at (-37.1333, 190.9333, 0) makes body 77 at (-37.1333, 200.9333, 0) makes body 78 at (-37.1333, 210.9333, 0) makes body 79 at (-37.1333, 220.9333, 0) makes body 80 at (-37.1333, 230.9333, 0) makes body 81 at (-37.1333, 240.9333, 0) makes body 82 at (-47.1333, 90.9333, 0) makes body 83 at (-47.1333, 100.9333, 0) makes body 84 at (-47.1333, 110.9333, 0) makes body 85 at (-47.1333, 120.9333, 0) makes body 86 at (-47.1333, 130.9333, 0) makes body 87 at (-47.1333, 140.9333, 0) makes body 88 at (-47.1333, 150.9333, 0) makes body 89 at (-47.1333, 160.9333, 0) makes body 90 at (-47.1333, 170.9333, 0) makes body 91 at (-47.1333, 180.9333, 0) makes body 92 at (-47.1333, 190.9333, 0) makes body 93 at (-47.1333, 200.9333, 0) makes body 94 at (-47.1333, 210.9333, 0) makes body 95 at (-47.1333, 220.9333, 0) makes body 96 at (-47.1333, 230.9333, 0) makes body 97 at (-47.1333, 240.9333, 0) makes body 98 at (-57.1333, 90.9333, 0) makes body 99 at (-57.1333, 100.9333, 0) makes body 100 at (-57.1333, 110.9333, 0) makes body 101 at (-57.1333, 120.9333, 0) makes body 102 at (-57.1333, 130.9333, 0) makes body 103 at (-57.1333, 140.9333, 0) makes body 104 at (-57.1333, 150.9333, 0) makes body 105 at (-57.1333, 160.9333, 0) makes body 106 at (-57.1333, 170.9333, 0) makes body 107 at (-57.1333, 180.9333, 0) makes body 108 at (-57.1333, 190.9333, 0) makes body 109 at (-57.1333, 200.9333, 0) makes body 110 at (-57.1333, 210.9333, 0) makes body 111 at (-57.1333, 220.9333, 0) makes body 112 at (-57.1333, 230.9333, 0) makes body 113 at (-57.1333, 240.9333, 0) makes body 114 at (-67.1333, 90.9333, 0) makes body 115 at (-67.1333, 100.9333, 0) makes body 116 at (-67.1333, 110.9333, 0) makes body 117 at (-67.1333, 120.9333, 0) makes body 118 at (-67.1333, 130.9333, 0) makes body 119 at (-67.1333, 140.9333, 0) makes body 120 at (-67.1333, 150.9333, 0) makes body 121 at (-67.1333, 160.9333, 0) makes body 122 at (-67.1333, 170.9333, 0) makes body 123 at (-67.1333, 180.9333, 0) makes body 124 at (-67.1333, 190.9333, 0) makes body 125 at (-67.1333, 200.9333, 0) makes body 126 at (-67.1333, 210.9333, 0) makes body 127 at (-67.1333, 220.9333, 0) makes body 128 at (-67.1333, 230.9333, 0) makes body 129 at (-67.1333, 240.9333, 0)
move_body "Desplazar1" bodies 1 to x (1, 0, 0) y (0, 1, 0) z (0, 0, 1) at (30, 0, 0)
move_body "Desplazar2" bodies 1 to x (0, 1, 0) y (-1, 0, 0) z (0, 0, 1) at (191, -191, 0)
move_body "Desplazar3" bodies 1 to x (1, 0, 0) y (0, 1, 0) z (0, 0, 1) at (-70, 250, 0)
sketch "Boceto14" plane through (0, 0, 0) normal (0, 0, -1) x (1, 0, 0)
  line L0 (110, -170) -> (110, -179)
  line L1 (110, -179) -> (101, -179)
  line L2 (101, -179) -> (101, -170)
  line L3 (101, -170) -> (110, -170)
  line L4 (110, -180) -> (110, -189)
  line L5 (110, -189) -> (101, -189)
  line L6 (101, -189) -> (101, -180)
  line L7 (101, -180) -> (110, -180)
  line L8 (110, -190) -> (110, -199)
  line L9 (110, -199) -> (101, -199)
  line L10 (101, -199) -> (101, -190)
  line L11 (101, -190) -> (110, -190)
  line L12 (110, -200) -> (110, -209)
  line L13 (110, -209) -> (101, -209)
  line L14 (101, -209) -> (101, -200)
  line L15 (101, -200) -> (110, -200)
  line L16 (110, -210) -> (110, -219)
  line L17 (110, -219) -> (101, -219)
  line L18 (101, -219) -> (101, -210)
  line L19 (101, -210) -> (110, -210)
  line L20 (110, -220) -> (110, -229)
  line L21 (110, -229) -> (101, -229)
  line L22 (101, -229) -> (101, -220)
  line L23 (101, -220) -> (110, -220)
  line L24 (100, -110) -> (100, -119)
  line L25 (100, -119) -> (91, -119)
  line L26 (91, -119) -> (91, -110)
  line L27 (91, -110) -> (100, -110)
  line L28 (110, -230) -> (110, -239)
  line L29 (110, -239) -> (101, -239)
  line L30 (101, -239) -> (101, -230)
  line L31 (101, -230) -> (110, -230)
  line L32 (110, -160) -> (110, -169)
  line L33 (110, -169) -> (101, -169)
  line L34 (101, -169) -> (101, -160)
  line L35 (101, -160) -> (110, -160)
  line L36 (110, -150) -> (110, -159)
  line L37 (110, -159) -> (101, -159)
  line L38 (101, -159) -> (101, -150)
  line L39 (101, -150) -> (110, -150)
  line L40 (110, -140) -> (110, -149)
  line L41 (110, -149) -> (101, -149)
  line L42 (101, -149) -> (101, -140)
  line L43 (101, -140) -> (110, -140)
  line L44 (110, -130) -> (110, -139)
  line L45 (110, -139) -> (101, -139)
  line L46 (101, -139) -> (101, -130)
  line L47 (101, -130) -> (110, -130)
  line L48 (110, -120) -> (110, -129)
  line L49 (110, -129) -> (101, -129)
  line L50 (101, -129) -> (101, -120)
  line L51 (101, -120) -> (110, -120)
  line L52 (110, -110) -> (110, -119)
  line L53 (110, -119) -> (101, -119)
  line L54 (101, -119) -> (101, -110)
  line L55 (101, -110) -> (110, -110)
  line L56 (110, -100) -> (110, -109)
  line L57 (110, -109) -> (101, -109)
  line L58 (101, -109) -> (101, -100)
  line L59 (101, -100) -> (110, -100)
  line L60 (100, -100) -> (100, -109)
  line L61 (100, -109) -> (91, -109)
  line L62 (91, -109) -> (91, -100)
  line L63 (91, -100) -> (100, -100)
  line L64 (110, -240) -> (110, -249)
  line L65 (110, -249) -> (101, -249)
  line L66 (101, -249) -> (101, -240)
  line L67 (101, -240) -> (110, -240)
  line L68 (100, -90) -> (100, -99)
  line L69 (100, -99) -> (91, -99)
  line L70 (91, -99) -> (91, -90)
  line L71 (91, -90) -> (100, -90)
  line L72 (120, -100) -> (120, -109)
  line L73 (120, -109) -> (111, -109)
  line L74 (111, -109) -> (111, -100)
  line L75 (111, -100) -> (120, -100)
  line L76 (100, -120) -> (100, -129)
  line L77 (100, -129) -> (91, -129)
  line L78 (91, -129) -> (91, -120)
  line L79 (91, -120) -> (100, -120)
  line L80 (100, -130) -> (100, -139)
  line L81 (100, -139) -> (91, -139)
  line L82 (91, -139) -> (91, -130)
  line L83 (91, -130) -> (100, -130)
  line L84 (100, -140) -> (100, -149)
  line L85 (100, -149) -> (91, -149)
  line L86 (91, -149) -> (91, -140)
  line L87 (91, -140) -> (100, -140)
  line L88 (100, -150) -> (100, -159)
  line L89 (100, -159) -> (91, -159)
  line L90 (91, -159) -> (91, -150)
  line L91 (91, -150) -> (100, -150)
  line L92 (100, -160) -> (100, -169)
  line L93 (100, -169) -> (91, -169)
  line L94 (91, -169) -> (91, -160)
  line L95 (91, -160) -> (100, -160)
  line L96 (100, -170) -> (100, -179)
  line L97 (100, -179) -> (91, -179)
  line L98 (91, -179) -> (91, -170)
  line L99 (91, -170) -> (100, -170)
  line L100 (100, -180) -> (100, -189)
  line L101 (100, -189) -> (91, -189)
  line L102 (91, -189) -> (91, -180)
  line L103 (91, -180) -> (100, -180)
  line L104 (100, -190) -> (100, -199)
  line L105 (100, -199) -> (91, -199)
  line L106 (91, -199) -> (91, -190)
  line L107 (91, -190) -> (100, -190)
  line L108 (100, -200) -> (100, -209)
  line L109 (100, -209) -> (91, -209)
  line L110 (91, -209) -> (91, -200)
  line L111 (91, -200) -> (100, -200)
  line L112 (100, -210) -> (100, -219)
  line L113 (100, -219) -> (91, -219)
  line L114 (91, -219) -> (91, -210)
  line L115 (91, -210) -> (100, -210)
  line L116 (100, -220) -> (100, -229)
  line L117 (100, -229) -> (91, -229)
  line L118 (91, -229) -> (91, -220)
  line L119 (91, -220) -> (100, -220)
  line L120 (100, -230) -> (100, -239)
  line L121 (100, -239) -> (91, -239)
  line L122 (91, -239) -> (91, -230)
  line L123 (91, -230) -> (100, -230)
  line L124 (100, -240) -> (100, -249)
  line L125 (100, -249) -> (91, -249)
  line L126 (91, -249) -> (91, -240)
  line L127 (91, -240) -> (100, -240)
  line L128 (90, -90) -> (90, -99)
  line L129 (90, -99) -> (81, -99)
  line L130 (81, -99) -> (81, -90)
  line L131 (81, -90) -> (90, -90)
  line L132 (90, -100) -> (90, -109)
  line L133 (90, -109) -> (81, -109)
  line L134 (81, -109) -> (81, -100)
  line L135 (81, -100) -> (90, -100)
  line L136 (90, -110) -> (90, -119)
  line L137 (90, -119) -> (81, -119)
  line L138 (81, -119) -> (81, -110)
  line L139 (81, -110) -> (90, -110)
  line L140 (90, -120) -> (90, -129)
  line L141 (90, -129) -> (81, -129)
  line L142 (81, -129) -> (81, -120)
  line L143 (81, -120) -> (90, -120)
  line L144 (90, -130) -> (90, -139)
  line L145 (90, -139) -> (81, -139)
  line L146 (81, -139) -> (81, -130)
  line L147 (81, -130) -> (90, -130)
  line L148 (90, -140) -> (90, -149)
  line L149 (90, -149) -> (81, -149)
  line L150 (81, -149) -> (81, -140)
  line L151 (81, -140) -> (90, -140)
  line L152 (90, -150) -> (90, -159)
  line L153 (90, -159) -> (81, -159)
  line L154 (81, -159) -> (81, -150)
  line L155 (81, -150) -> (90, -150)
  line L156 (90, -160) -> (90, -169)
  line L157 (90, -169) -> (81, -169)
  line L158 (81, -169) -> (81, -160)
  line L159 (81, -160) -> (90, -160)
  line L160 (90, -170) -> (90, -179)
  line L161 (90, -179) -> (81, -179)
  line L162 (81, -179) -> (81, -170)
  line L163 (81, -170) -> (90, -170)
  line L164 (90, -180) -> (90, -189)
  line L165 (90, -189) -> (81, -189)
  line L166 (81, -189) -> (81, -180)
  line L167 (81, -180) -> (90, -180)
  line L168 (90, -190) -> (90, -199)
  line L169 (90, -199) -> (81, -199)
  line L170 (81, -199) -> (81, -190)
  line L171 (81, -190) -> (90, -190)
  line L172 (90, -200) -> (90, -209)
  line L173 (90, -209) -> (81, -209)
  line L174 (81, -209) -> (81, -200)
  line L175 (81, -200) -> (90, -200)
  line L176 (90, -210) -> (90, -219)
  line L177 (90, -219) -> (81, -219)
  line L178 (81, -219) -> (81, -210)
  line L179 (81, -210) -> (90, -210)
  line L180 (90, -220) -> (90, -229)
  line L181 (90, -229) -> (81, -229)
  line L182 (81, -229) -> (81, -220)
  line L183 (81, -220) -> (90, -220)
  line L184 (90, -230) -> (90, -239)
  line L185 (90, -239) -> (81, -239)
  line L186 (81, -239) -> (81, -230)
  line L187 (81, -230) -> (90, -230)
  line L188 (90, -240) -> (90, -249)
  line L189 (90, -249) -> (81, -249)
  line L190 (81, -249) -> (81, -240)
  line L191 (81, -240) -> (90, -240)
  line L192 (80, -90) -> (80, -99)
  line L193 (80, -99) -> (71, -99)
  line L194 (71, -99) -> (71, -90)
  line L195 (71, -90) -> (80, -90)
  line L196 (80, -100) -> (80, -109)
  line L197 (80, -109) -> (71, -109)
  line L198 (71, -109) -> (71, -100)
  line L199 (71, -100) -> (80, -100)
  line L200 (80, -110) -> (80, -119)
  line L201 (80, -119) -> (71, -119)
  line L202 (71, -119) -> (71, -110)
  line L203 (71, -110) -> (80, -110)
  line L204 (80, -120) -> (80, -129)
  line L205 (80, -129) -> (71, -129)
  line L206 (71, -129) -> (71, -120)
  line L207 (71, -120) -> (80, -120)
  line L208 (80, -130) -> (80, -139)
  line L209 (80, -139) -> (71, -139)
  line L210 (71, -139) -> (71, -130)
  line L211 (71, -130) -> (80, -130)
  line L212 (80, -140) -> (80, -149)
  line L213 (80, -149) -> (71, -149)
  line L214 (71, -149) -> (71, -140)
  line L215 (71, -140) -> (80, -140)
  line L216 (80, -150) -> (80, -159)
  line L217 (80, -159) -> (71, -159)
  line L218 (71, -159) -> (71, -150)
  line L219 (71, -150) -> (80, -150)
  line L220 (80, -160) -> (80, -169)
  line L221 (80, -169) -> (71, -169)
  line L222 (71, -169) -> (71, -160)
  line L223 (71, -160) -> (80, -160)
  line L224 (80, -170) -> (80, -179)
  line L225 (80, -179) -> (71, -179)
  line L226 (71, -179) -> (71, -170)
  line L227 (71, -170) -> (80, -170)
  line L228 (80, -180) -> (80, -189)
  line L229 (80, -189) -> (71, -189)
  line L230 (71, -189) -> (71, -180)
  line L231 (71, -180) -> (80, -180)
  line L232 (80, -190) -> (80, -199)
  line L233 (80, -199) -> (71, -199)
  line L234 (71, -199) -> (71, -190)
  line L235 (71, -190) -> (80, -190)
  line L236 (80, -200) -> (80, -209)
  line L237 (80, -209) -> (71, -209)
  line L238 (71, -209) -> (71, -200)
  line L239 (71, -200) -> (80, -200)
  line L240 (80, -210) -> (80, -219)
  line L241 (80, -219) -> (71, -219)
  line L242 (71, -219) -> (71, -210)
  line L243 (71, -210) -> (80, -210)
  line L244 (80, -220) -> (80, -229)
  line L245 (80, -229) -> (71, -229)
  line L246 (71, -229) -> (71, -220)
  line L247 (71, -220) -> (80, -220)
  line L248 (80, -230) -> (80, -239)
  line L249 (80, -239) -> (71, -239)
  line L250 (71, -239) -> (71, -230)
  line L251 (71, -230) -> (80, -230)
  line L252 (80, -240) -> (80, -249)
  line L253 (80, -249) -> (71, -249)
  line L254 (71, -249) -> (71, -240)
  line L255 (71, -240) -> (80, -240)
  line L256 (70, -90) -> (70, -99)
  line L257 (70, -99) -> (61, -99)
  line L258 (61, -99) -> (61, -90)
  line L259 (61, -90) -> (70, -90)
  line L260 (70, -100) -> (70, -109)
  line L261 (70, -109) -> (61, -109)
  line L262 (61, -109) -> (61, -100)
  line L263 (61, -100) -> (70, -100)
  line L264 (70, -110) -> (70, -119)
  line L265 (70, -119) -> (61, -119)
  line L266 (61, -119) -> (61, -110)
  line L267 (61, -110) -> (70, -110)
  line L268 (70, -120) -> (70, -129)
  line L269 (70, -129) -> (61, -129)
  line L270 (61, -129) -> (61, -120)
  line L271 (61, -120) -> (70, -120)
  line L272 (70, -130) -> (70, -139)
  line L273 (70, -139) -> (61, -139)
  line L274 (61, -139) -> (61, -130)
  line L275 (61, -130) -> (70, -130)
  line L276 (70, -140) -> (70, -149)
  line L277 (70, -149) -> (61, -149)
  line L278 (61, -149) -> (61, -140)
  line L279 (61, -140) -> (70, -140)
  line L280 (70, -150) -> (70, -159)
  line L281 (70, -159) -> (61, -159)
  line L282 (61, -159) -> (61, -150)
  line L283 (61, -150) -> (70, -150)
  line L284 (70, -160) -> (70, -169)
  line L285 (70, -169) -> (61, -169)
  line L286 (61, -169) -> (61, -160)
  line L287 (61, -160) -> (70, -160)
  line L288 (70, -170) -> (70, -179)
  line L289 (70, -179) -> (61, -179)
  line L290 (61, -179) -> (61, -170)
  line L291 (61, -170) -> (70, -170)
  line L292 (70, -180) -> (70, -189)
  line L293 (70, -189) -> (61, -189)
  line L294 (61, -189) -> (61, -180)
  line L295 (61, -180) -> (70, -180)
  line L296 (70, -190) -> (70, -199)
  line L297 (70, -199) -> (61, -199)
  line L298 (61, -199) -> (61, -190)
  line L299 (61, -190) -> (70, -190)
  line L300 (70, -200) -> (70, -209)
  line L301 (70, -209) -> (61, -209)
  line L302 (61, -209) -> (61, -200)
  line L303 (61, -200) -> (70, -200)
  line L304 (70, -210) -> (70, -219)
  line L305 (70, -219) -> (61, -219)
  line L306 (61, -219) -> (61, -210)
  line L307 (61, -210) -> (70, -210)
  line L308 (70, -220) -> (70, -229)
  line L309 (70, -229) -> (61, -229)
  line L310 (61, -229) -> (61, -220)
  line L311 (61, -220) -> (70, -220)
  line L312 (70, -230) -> (70, -239)
  line L313 (70, -239) -> (61, -239)
  line L314 (61, -239) -> (61, -230)
  line L315 (61, -230) -> (70, -230)
  line L316 (70, -240) -> (70, -249)
  line L317 (70, -249) -> (61, -249)
  line L318 (61, -249) -> (61, -240)
  line L319 (61, -240) -> (70, -240)
  line L320 (60, -90) -> (60, -99)
  line L321 (60, -99) -> (51, -99)
  line L322 (51, -99) -> (51, -90)
  line L323 (51, -90) -> (60, -90)
  line L324 (60, -100) -> (60, -109)
  line L325 (60, -109) -> (51, -109)
  line L326 (51, -109) -> (51, -100)
  line L327 (51, -100) -> (60, -100)
  line L328 (60, -110) -> (60, -119)
  line L329 (60, -119) -> (51, -119)
  line L330 (51, -119) -> (51, -110)
  line L331 (51, -110) -> (60, -110)
  line L332 (60, -120) -> (60, -129)
  line L333 (60, -129) -> (51, -129)
  line L334 (51, -129) -> (51, -120)
  line L335 (51, -120) -> (60, -120)
  line L336 (60, -130) -> (60, -139)
  line L337 (60, -139) -> (51, -139)
  line L338 (51, -139) -> (51, -130)
  line L339 (51, -130) -> (60, -130)
  line L340 (60, -140) -> (60, -149)
  line L341 (60, -149) -> (51, -149)
  line L342 (51, -149) -> (51, -140)
  line L343 (51, -140) -> (60, -140)
  line L344 (60, -150) -> (60, -159)
  line L345 (60, -159) -> (51, -159)
  line L346 (51, -159) -> (51, -150)
  line L347 (51, -150) -> (60, -150)
  line L348 (60, -160) -> (60, -169)
  line L349 (60, -169) -> (51, -169)
  line L350 (51, -169) -> (51, -160)
  line L351 (51, -160) -> (60, -160)
  line L352 (60, -170) -> (60, -179)
  line L353 (60, -179) -> (51, -179)
  line L354 (51, -179) -> (51, -170)
  line L355 (51, -170) -> (60, -170)
  line L356 (60, -180) -> (60, -189)
  line L357 (60, -189) -> (51, -189)
  line L358 (51, -189) -> (51, -180)
  line L359 (51, -180) -> (60, -180)
  line L360 (60, -190) -> (60, -199)
  line L361 (60, -199) -> (51, -199)
  line L362 (51, -199) -> (51, -190)
  line L363 (51, -190) -> (60, -190)
  line L364 (60, -200) -> (60, -209)
  line L365 (60, -209) -> (51, -209)
  line L366 (51, -209) -> (51, -200)
  line L367 (51, -200) -> (60, -200)
  line L368 (60, -210) -> (60, -219)
  line L369 (60, -219) -> (51, -219)
  line L370 (51, -219) -> (51, -210)
  line L371 (51, -210) -> (60, -210)
  line L372 (60, -220) -> (60, -229)
  line L373 (60, -229) -> (51, -229)
  line L374 (51, -229) -> (51, -220)
  line L375 (51, -220) -> (60, -220)
  line L376 (60, -230) -> (60, -239)
  line L377 (60, -239) -> (51, -239)
  line L378 (51, -239) -> (51, -230)
  line L379 (51, -230) -> (60, -230)
  line L380 (60, -240) -> (60, -249)
  line L381 (60, -249) -> (51, -249)
  line L382 (51, -249) -> (51, -240)
  line L383 (51, -240) -> (60, -240)
  line L384 (50, -90) -> (50, -99)
  line L385 (50, -99) -> (41, -99)
  line L386 (41, -99) -> (41, -90)
  line L387 (41, -90) -> (50, -90)
  line L388 (50, -100) -> (50, -109)
  line L389 (50, -109) -> (41, -109)
  line L390 (41, -109) -> (41, -100)
  line L391 (41, -100) -> (50, -100)
  line L392 (50, -110) -> (50, -119)
  line L393 (50, -119) -> (41, -119)
  line L394 (41, -119) -> (41, -110)
  line L395 (41, -110) -> (50, -110)
  line L396 (50, -120) -> (50, -129)
  line L397 (50, -129) -> (41, -129)
  line L398 (41, -129) -> (41, -120)
  line L399 (41, -120) -> (50, -120)
  line L400 (50, -130) -> (50, -139)
  line L401 (50, -139) -> (41, -139)
  line L402 (41, -139) -> (41, -130)
  line L403 (41, -130) -> (50, -130)
  line L404 (50, -140) -> (50, -149)
  line L405 (50, -149) -> (41, -149)
  line L406 (41, -149) -> (41, -140)
  line L407 (41, -140) -> (50, -140)
  line L408 (50, -150) -> (50, -159)
  line L409 (50, -159) -> (41, -159)
  line L410 (41, -159) -> (41, -150)
  line L411 (41, -150) -> (50, -150)
  line L412 (50, -160) -> (50, -169)
  line L413 (50, -169) -> (41, -169)
  line L414 (41, -169) -> (41, -160)
  line L415 (41, -160) -> (50, -160)
  line L416 (50, -170) -> (50, -179)
  line L417 (50, -179) -> (41, -179)
  line L418 (41, -179) -> (41, -170)
  line L419 (41, -170) -> (50, -170)
  line L420 (50, -180) -> (50, -189)
  line L421 (50, -189) -> (41, -189)
  line L422 (41, -189) -> (41, -180)
  line L423 (41, -180) -> (50, -180)
  line L424 (50, -190) -> (50, -199)
  line L425 (50, -199) -> (41, -199)
  line L426 (41, -199) -> (41, -190)
  line L427 (41, -190) -> (50, -190)
  line L428 (50, -200) -> (50, -209)
  line L429 (50, -209) -> (41, -209)
  line L430 (41, -209) -> (41, -200)
  line L431 (41, -200) -> (50, -200)
  line L432 (50, -210) -> (50, -219)
  line L433 (50, -219) -> (41, -219)
  line L434 (41, -219) -> (41, -210)
  line L435 (41, -210) -> (50, -210)
  line L436 (50, -220) -> (50, -229)
  line L437 (50, -229) -> (41, -229)
  line L438 (41, -229) -> (41, -220)
  line L439 (41, -220) -> (50, -220)
  line L440 (50, -230) -> (50, -239)
  line L441 (50, -239) -> (41, -239)
  line L442 (41, -239) -> (41, -230)
  line L443 (41, -230) -> (50, -230)
  line L444 (50, -240) -> (50, -249)
  line L445 (50, -249) -> (41, -249)
  line L446 (41, -249) -> (41, -240)
  line L447 (41, -240) -> (50, -240)
  line L448 (120, -240) -> (120, -249)
  line L449 (120, -249) -> (111, -249)
  line L450 (111, -249) -> (111, -240)